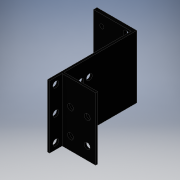
# Autodesk Inventor part: TrolleyRightPlate
Saved by Autodesk Inventor 2016 (Build 200138000, 138)
## iProperties
Created: 2016-03-27
Part Number: TrolleyRightPlate
Material: UHMW, Black
Document SubType Name: Modeling
Designer: mkepler
Density: 0.94 g/cm^3
Appearance: Smooth - Black
Mass: 7.99184 g
Surface Area: 106.873 cm^2
Volume: 8.50196 cm^3
Author: mkepler
Autodesk Inventor part; units mm, degrees
ref_plane "YZ Plane" through (0, 0, 0) normal (1, 0, 0) x (0, 1, 0)
ref_plane "XZ Plane" through (0, 0, 0) normal (0, 1, 0) x (-1, 0, 0)
ref_plane "XY Plane" through (0, 0, 0) normal (0, 0, 1) x (1, 0, 0)
sketch "Sketch3" plane through (0, 0, 0) normal (0, 1, 0) x (-1, 0, 0)
  line L0 (0, 0) -> (27, 0)
  line L1 (27, 0) -> (27, -45)
  line L2 (27, -45) -> (0, -45)
  line L3 (0, -45) -> (0, 0)
  dimension "d27" = 27
  dimension "d28" = 45
  constraints: 8 end point, 2 parallel, 1 horizontal, 1 perpendicular
  measures "d27" distance of L1.end L2.end
  measures "d28" distance of L0.end L1.end
extrude "Extrusion2" add sketch "Sketch3" along normal blind 2.5
sketch "Sketch4" plane through (0, 0, 0) normal (0, -1, 0) x (1, 0, 0)
  line L0 (0, 0) -> (1.5, 0)
  line L1 (1.5, 0) -> (1.5, -45)
  line L2 (1.5, -45) -> (0, -45)
  line L3 (0, -45) -> (0, 0)
  dimension "d31" = 1.5
  dimension "d32" = 45
  constraints: 8 end point, 2 parallel, 1 horizontal, 1 perpendicular
  measures "d31" distance of L1.end L2.end
  measures "d32" distance of L0.end L1.end
extrude "Extrusion3" add sketch "Sketch4" along normal blind 60 and the other way blind 2.5
sketch "Sketch5" plane through (0, 2.5, 0) normal (0, 1, 0) x (1, 0, 0)
  line L0 (-27, 0) -> (-27, 45) projected
  line L1 (-27, 0) -> (1.5, 0) projected
  circle A0 centre (-3.5, 3.5) radius 2.3
  line L2 (0, 45) -> (0, 0) projected
  circle A1 centre (-23.5, 41.5) radius 2.3
  line L3 (1.5, 45) -> (-27, 45) projected
  circle A2 centre (-3.5, 41.5) radius 2.3
  dimension "d45" = 4.6
  dimension "d46" = 3.5
  dimension "d47" = 3.5
  dimension "d50" = 4.6
  dimension "d51" = 3.5
  dimension "d52" = 4.6
  dimension "d61" = 3.5
  dimension "d62" = 3.5
  dimension "d63" = 3.5
  constraints: 3 centre point
  measures "d45" diameter of A0
  measures "d46" distance from line of A0.centre L2
  measures "d47" distance from line of L1 A0.centre
  measures "d50" diameter of A1
  measures "d51" distance from line of L3 A1.centre
  measures "d52" diameter of A2
  measures "d61" distance from line of L0 A1.centre
  measures "d62" distance from line of L3 A2.centre
  measures "d63" distance from line of L2 A2.centre
hole "Hole2" at (-3.5, 2.5, -3.5) at (-3.5, 2.5, -41.5) at (-23.5, 2.5, -41.5) direction (0, -1, 0) diameter 4.6 end through all
sketch "Sketch6" plane through (0, 2.5, 0) normal (0, 1, 0) x (1, 0, 0)
  circle A0 centre (-21, 7.5) radius 1.5
  line L0 (-27, 45) -> (-27, 0) projected
  line L1 (-27, 0) -> (1.5, 0) projected
  circle A1 centre (-21, 25.5) radius 1.5
  point P0 (0, 0)
  dimension "d64" = 3
  dimension "d65" = 6
  dimension "d66" = 7.5
  dimension "d67" = 3
  dimension "d68" = 18
  constraints: 2 centre point
  measures "d64" diameter of A0
  measures "d65" distance from line of A0.centre L0
  measures "d66" distance from line of L1 A0.centre
  measures "d67" diameter of A1
  measures "d68" distance of A1.centre A0.centre
hole "Hole3" at (-21, 2.5, -7.5) at (-21, 2.5, -25.5) direction (0, -1, 0) diameter 3 end through all
sketch "Sketch7" plane through (1.5, -60, 0) normal (1, 0, 0) x (0, 0, -1)
  circle A0 centre (4.5, 4.5) radius 2.15
  line L0 (45, 0) -> (0, 0) projected
  line L1 (0, 0) -> (0, 62.5) projected
  circle A1 centre (40.5, 4.5) radius 2.15
  line L2 (45, 0) -> (45, 62.5) projected
  circle A2 centre (22.5, 4.5) radius 2.15
  point P0 (0, 60)
  dimension "d76" = 4.3
  dimension "d77" = 4.5
  dimension "d78" = 4.5
  dimension "d79" = 4.3
  dimension "d80" = 4.5
  dimension "d81" = 4.5
  dimension "d82" = 4.3
  constraints: 3 centre point
  measures "d76" diameter of A0
  measures "d77" distance from line of A0.centre L0
  measures "d78" distance from line of L1 A0.centre
  measures "d79" diameter of A1
  measures "d80" distance from line of A1.centre L2
  measures "d81" distance from line of L0 A1.centre
  measures "d82" diameter of A2
hole "Hole4" at (1.5, -55.5, -4.5) at (1.5, -55.5, -22.5) at (1.5, -55.5, -40.5) direction (-1, 0, 0) diameter 4.3 end through all
sketch "Sketch8" plane through (1.5, -60, 0) normal (1, 0, 0) x (0, 0, -1)
  line L0 (0, 9) -> (45, 9)
  line L1 (45, 9) -> (45, 10.5)
  line L2 (45, 10.5) -> (0, 10.5)
  line L3 (0, 10.5) -> (0, 9)
  line L4 (0, 62.5) -> (45, 62.5) projected
  point P0 (0, 60)
  dimension "d90" = 45
  dimension "d91" = 1.5
  dimension "d92" = 52
  constraints: 8 end point, 2 parallel, 1 horizontal, 1 perpendicular
  measures "d90" distance of L2.end L1.end
  measures "d91" distance of L1.end L0.end
  measures "d92" distance between parallel lines of L2 L4
extrude "Extrusion4" add sketch "Sketch8" along normal blind 24
sketch "Sketch10" plane through (1.5, -49.5, 0) normal (0, 1, 0) x (1, 0, 0)
  circle A0 centre (6, 36) radius 2.125
  line L0 (0, 45) -> (24, 45) projected
  line L1 (0, 0) -> (0, 45) projected
  circle A1 centre (18, 36) radius 2.125
  line L2 (6, 36) -> (6, 27)
  line L3 (6, 27) -> (12, 27)
  circle A2 centre (6, 18) radius 2.125
  circle A3 centre (18, 18) radius 2.125
  point P0 (-1.5, 0)
  dimension "d95" = 4.25
  dimension "d96" = 9
  dimension "d97" = 6
  dimension "d100" = 4.25
  dimension "d102" = 9
  constraints: 4 centre point, 4 end point, 2 symmetric about line, 1 perpendicular, 1 vertical, 2 other
  measures "d95" diameter of A0
  measures "d96" distance from line of L0 L2.start
  measures "d97" distance from line of L1 L2.start
  measures "d100" diameter of A1
  measures "d102" distance of L2.start L2.end
hole "Hole6" at (7.5, -49.5, -18) at (7.5, -49.5, -36) at (19.5, -49.5, -36) at (19.5, -49.5, -18) direction (0, -1, 0) diameter 4.25 end through all
sketch "Sketch11" plane through (1.5, 2.5, 0) normal (1, 0, 0) x (0, 0, -1)
  circle A0 centre (12, -46) radius 2.125
  line L0 (45, -52) -> (45, 0) projected
  line L1 (0, -52) -> (0, 0) projected
  line L2 (0, -52) -> (45, -52) projected
  circle A1 centre (12, -40) radius 2.125
  circle A2 centre (12, -34) radius 2.125
  point P0 (0, -2.5)
  dimension "d117" = 4.25
  dimension "d119" = 12
  dimension "d120" = 6
  dimension "d121" = 4.25
  dimension "d122" = 6
  dimension "d123" = 4.25
  dimension "d124" = 6
  constraints: 3 centre point
  measures "d117" diameter of A0
  measures "d119" distance from line of L1 A0.centre
  measures "d120" distance from line of A0.centre L2
  measures "d121" diameter of A1
  measures "d122" distance of A1.centre A0.centre
  measures "d123" diameter of A2
  measures "d124" distance of A1.centre A2.centre
hole "Hole7" at (1.5, -31.5, -12) at (1.5, -37.5, -12) at (1.5, -43.5, -12) direction (-1, 0, 0) diameter 4.25 depth 8 tip angle 118
body "Solid2"
